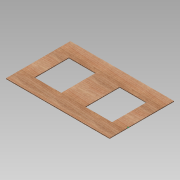
# Autodesk Inventor part: cart_woodpanel-back
Saved by Autodesk Inventor 2015 (Build 190159000, 159)
## iProperties
Created: 2015-05-21
Part Number: cart_woodpanel-back
Material: Wood (Birch)
Document SubType Name: Modeling
Designer: Joe Sheldon
Density: 0.55 g/cm^3
Appearance: Birch - Natural Polished
Author: Joe Sheldon
Autodesk Inventor part; units mm, degrees
ref_plane "YZ Plane" through (0, 0, 0) normal (1, 0, 0) x (0, 1, 0)
ref_plane "XZ Plane" through (0, 0, 0) normal (0, 1, 0) x (-1, 0, 0)
ref_plane "XY Plane" through (0, 0, 0) normal (0, 0, 1) x (1, 0, 0)
sketch "Sketch1" plane through (0, 0, 0) normal (0, 1, 0) x (-1, 0, 0)
  line L0 (0, 0) -> (685.8, 0)
  line L1 (685.8, 0) -> (685.8, -304.8)
  line L2 (685.8, -304.8) -> (0, -304.8)
  line L3 (0, -304.8) -> (0, 0)
  line L4 (685.8, 0) -> (0, 0)
  line L5 (0, 0) -> (0, 120.65)
  line L6 (0, 120.65) -> (685.8, 120.65)
  line L7 (685.8, 120.65) -> (685.8, 0)
  dimension "d0" = 685.8
  dimension "d1" = 304.8
  dimension "d4" = 120.65
  constraints: 16 end point, 4 parallel, 2 horizontal, 2 perpendicular
  measures "d0" distance of L1.end L2.end
  measures "d1" distance of L0.end L1.end
  measures "d4" distance of L4.end L5.end
extrude "Extrusion1" add sketch "Sketch1" along normal blind 5.08 contours L0 L1 L2 L3
sketch "Sketch2" plane through (-685.8, 0, 0) normal (0, 0, 1) x (1, 0, 0)
  line L0 (685.8, 0) -> (0, 0) projected
  line L1 (685.8, 0) -> (685.8, 5.08) projected
  line L2 (0, 5.08) -> (685.8, 5.08) projected
  line L3 (0, 0) -> (0, 5.08) projected
extrude "Extrusion2" add sketch "Sketch2" along normal blind 120.65
sketch "Sketch3" plane through (0, 5.08, 0) normal (0, 1, 0) x (1, 0, 0)
  point P0 (0, 0)
sketch "Sketch4" plane through (0, 5.08, 0) normal (0, 1, 0) x (1, 0, 0)
  line L0 (-685.8, -120.65) -> (-685.8, 304.8) projected
  line L1 (-685.8, 92.075) -> (-609.6, 92.075)
  line L2 (-609.6, 92.075) -> (-609.6, -34.925)
  line L3 (-609.6, 92.075) -> (-609.6, 219.075)
  line L4 (-609.6, 219.075) -> (-406.4, 219.075)
  line L5 (-406.4, 219.075) -> (-406.4, -34.925)
  line L6 (-406.4, -34.925) -> (-609.6, -34.925)
  line L7 (0, 304.8) -> (0, -120.65) projected
  line L8 (0, 92.075) -> (-69.85, 92.075)
  line L9 (-69.85, 92.075) -> (-69.85, 219.075)
  line L10 (-69.85, 219.075) -> (-273.05, 219.075)
  line L11 (-273.05, 219.075) -> (-273.05, -34.925)
  line L12 (-273.05, -34.925) -> (-69.85, -34.925)
  line L13 (-69.85, -34.925) -> (-69.85, 92.075)
  line L14 (-419.1, -22.225) -> (-419.1, 206.375)
  line L15 (-419.1, 206.375) -> (-596.9, 206.375)
  line L16 (-596.9, 206.375) -> (-596.9, 92.075)
  line L17 (-596.9, 92.075) -> (-596.9, -22.225)
  line L18 (-596.9, -22.225) -> (-419.1, -22.225)
  line L19 (-260.35, -22.225) -> (-260.35, 206.375)
  line L20 (-260.35, 206.375) -> (-82.55, 206.375)
  line L21 (-82.55, 206.375) -> (-82.55, 92.075)
  line L22 (-82.55, 92.075) -> (-82.55, -22.225)
  line L23 (-82.55, -22.225) -> (-260.35, -22.225)
  point P0 (0, 0)
  dimension "d7" = 76.2
  dimension "d8" = 127
  dimension "d9" = 127
  dimension "d10" = 203.2
  dimension "d11" = 69.85
  dimension "d12" = 203.2
  dimension "d13" = 12.7
  dimension "d14" = 12.7
  constraints: 44 end point, 13 perpendicular, 3 horizontal, 2 midpoint, 2 vertical, 1 point on line, 8 other
  measures "d7" distance of L1.start L1.end
  measures "d8" distance of L1.end L2.end
  measures "d9" distance of L1.end L3.end
  measures "d10" distance of L3.end L4.end
  measures "d11" distance of L8.start L8.end
  measures "d12" distance of L9.end L10.end
  measures "d13" distance between parallel lines of L5 L14
  measures "d14" distance between parallel lines of L11 L19
extrude "Extrusion3" cut sketch "Sketch4" against normal blind 25.4 contours L18 L17 L16 L15 L14 | L19 L20 L21 L22 L23
sketch "Sketch5" plane through (0, 5.08, 0) normal (0, 1, 0) x (1, 0, 0)
  point P0 (0, 0)
body "Solid1"
